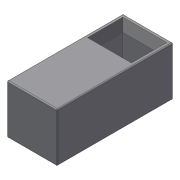
# Autodesk Inventor part: box
Saved by Autodesk Inventor 2014 (Build 180170000, 170)
## iProperties
Created: 2014-05-05
Part Number: box
Material: 一般
Document SubType Name: Modeling
Designer: motegi
Density: 1 g/cm^3
Appearance: 既定
Author: motegi
Autodesk Inventor part; units mm, degrees
ref_plane "YZ Plane" through (0, 0, 0) normal (1, 0, 0) x (0, 1, 0)
ref_plane "XZ Plane" through (0, 0, 0) normal (0, 1, 0) x (-1, 0, 0)
ref_plane "XY Plane" through (0, 0, 0) normal (0, 0, 1) x (1, 0, 0)
sketch "スケッチ1" plane through (0, 0, 0) normal (0, 1, 0) x (-1, 0, 0)
  line L0 (241, -236) -> (-241, -236)
  line L1 (-241, -236) -> (-241, 236)
  line L2 (-241, 236) -> (241, 236)
  line L3 (241, 236) -> (241, -236)
  line L4 (241, -236) -> (-241, 236) construction
  line L5 (-241, -236) -> (241, 236) construction
  point P0 (0, 0)
  dimension "d0" = 482
  dimension "d1" = 472
  constraints: 12 end point, 2 midpoint, 2 parallel, 1 horizontal, 1 perpendicular
  measures "d0" distance of L1.end L2.end
  measures "d1" distance of L0.end L1.end
extrude "押し出し1" add sketch "スケッチ1" along normal blind 1113
fillet "フィレット1" radius 10 12 edges at (241, 1113, 0) (0, 1113, -236) (-241, 1113, 0) (0, 1113, 236) (-241, 556.5, 236) (241, 556.5, 236) (241, 556.5, -236) (-241, 556.5, -236) (0, 0, 236) (-241, 0, 0) (0, 0, -236) (241, 0, 0)
sketch "スケッチ2" plane through (0, 1113, 0) normal (0, 1, 0) x (1, 0, 0)
  line L0 (-212, -205) -> (212, -205)
  line L1 (212, -205) -> (212, 205)
  line L2 (212, 205) -> (-212, 205)
  line L3 (-212, 205) -> (-212, -205)
  line L4 (-212, -205) -> (212, 205) construction
  line L5 (212, -205) -> (-212, 205) construction
  point P0 (0, 0)
  dimension "d5" = 424
  dimension "d6" = 410
  constraints: 12 end point, 2 midpoint, 2 parallel, 1 horizontal, 1 perpendicular
  measures "d5" distance of L2.end L1.end
  measures "d6" distance of L1.end L0.end
extrude "押し出し2" cut sketch "スケッチ2" against normal blind 1.45
sketch "スケッチ3" plane through (-231, 1103, 236) normal (0, 0, 1) x (1, 0, 0)
  line L0 (20, -20) -> (442, -20)
  line L1 (442, -20) -> (442, -360)
  line L2 (442, -360) -> (20, -360)
  line L3 (20, -360) -> (20, -20)
  point P0 (231, -1103)
  dimension "d9" = 422
  dimension "d10" = 340
  constraints: 8 end point, 2 parallel, 1 horizontal, 1 perpendicular
  measures "d9" distance of L1.end L2.end
  measures "d10" distance of L0.end L1.end
extrude "押し出し3" cut sketch "スケッチ3" against normal blind 100
draft "面の勾配1" angle 15 pull direction (0, 0, 1) faces at (70.3333, 743, 202.6667) fixed edges at (0, 743, 236)
draft "面の勾配2" angle 15 pull direction (0, 0, 1) faces at (-211, 865.265, 202.6667) fixed edges at (-211, 913, 236)
draft "面の勾配3" angle 15 pull direction (0, 0, 1) faces at (-61.4017, 1083, 202.6667) fixed edges at (0, 1083, 236)
draft "面の勾配4" angle 15 pull direction (0, 0, 1) faces at (211, 865.265, 202.6667) fixed edges at (211, 913, 236)
sketch "スケッチ4" plane through (-231, 1103, 136) normal (0, 0, 1) x (1, 0, 0)
  line L0 (46.7949, -46.7949) -> (415.2051, -46.7949)
  line L1 (415.2051, -46.7949) -> (415.2051, -333.2051)
  line L2 (415.2051, -333.2051) -> (46.7949, -333.2051)
  line L3 (46.7949, -333.2051) -> (46.7949, -46.7949)
  point P0 (231, -1103)
  constraints: 8 end point, 2 parallel, 1 horizontal, 1 perpendicular
extrude "押し出し4" cut sketch "スケッチ4" against normal blind 343
